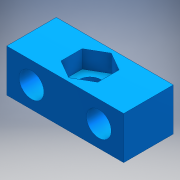
# Autodesk Inventor part: smallSprocketFixture
Saved by Autodesk Inventor 2016 (Build 200138000, 138)
## iProperties
Created: 2016-05-21
Part Number: smallSprocketFixture
Material: ABS Plastic
Document SubType Name: Modeling
Designer: Henrik Samuelsson
Density: 1.06 g/cm^3
Appearance: Smooth - White
Author: Henrik Samuelsson
Autodesk Inventor part; units mm, degrees
ref_plane "YZ Plane" through (0, 0, 0) normal (1, 0, 0) x (0, 1, 0)
ref_plane "XZ Plane" through (0, 0, 0) normal (0, 1, 0) x (-1, 0, 0)
ref_plane "XY Plane" through (0, 0, 0) normal (0, 0, 1) x (1, 0, 0)
sketch "Sketch1" plane through (0, 0, 0) normal (0, 1, 0) x (-1, 0, 0)
  line L0 (0, 0) -> (33, 0)
  line L1 (33, 0) -> (33, -12)
  line L2 (33, -12) -> (0, -12)
  line L3 (0, -12) -> (0, 0)
  circle A0 centre (26, -6) radius 3.5
  circle A1 centre (7, -6) radius 3.5
  dimension "d0" = 12
  dimension "d1" = 33
  dimension "d2" = 7
  dimension "d3" = 7
  dimension "d4" = 7
  dimension "d6" = 6
  dimension "d7" = 6
  dimension "d9" = 19
  constraints: 8 end point, 2 centre point, 2 parallel, 1 horizontal, 1 perpendicular
  measures "d0" distance of L1.end L0.end
  measures "d1" distance of L2.end L1.end
  measures "d2" diameter of A0
  measures "d3" diameter of A1
  measures "d4" distance from line of L1 A0.centre
  measures "d6" distance from line of L2 A1.centre
  measures "d7" distance from line of L2 A0.centre
  measures "d9" distance of A0.centre A1.centre
extrude "Extrusion1" add sketch "Sketch1" along normal mid plane 14
sketch "Sketch2" plane through (0, -7, -12) normal (0, 0, -1) x (-1, 0, 0)
  circle A0 centre (16.5, 7) radius 3.1
  line L0 (33, 14) -> (33, 0) projected
  line L1 (33, 0) -> (0, 0) projected
  point P0 (0, 7)
  dimension "d12" = 6.2
  dimension "d14" = 16.5
  dimension "d20" = 7
  constraints: 1 centre point
  measures "d12" diameter of A0
  measures "d14" distance from line of L0 A0.centre
  measures "d20" distance from line of L1 A0.centre
extrude "Extrusion2" cut sketch "Sketch2" against normal up to next
sketch "Sketch3" plane through (-33, -7, 0) normal (0, 0, 1) x (1, 0, 0)
  circle A0 centre (16.5, 7) radius 3.1 projected
  line L0 (16.5, 13.0044) -> (21.7, 10.0022)
  line L1 (21.7, 10.0022) -> (21.7, 3.9978)
  line L2 (21.7, 3.9978) -> (16.5, 0.9956)
  line L3 (16.5, 0.9956) -> (11.3, 3.9978)
  line L4 (11.3, 3.9978) -> (11.3, 10.0022)
  line L5 (11.3, 10.0022) -> (16.5, 13.0044)
  line L6 (0, 14) -> (33, 14) projected
  line L7 (0, 14) -> (0, 0) projected
  point P0 (33, 7)
  dimension "d17" = 5.2
  constraints: 12 end point, 1 coincident, 1 parallel, 12 other
  measures "d17" distance from line of L5 point (16.5, 7)
extrude "Extrusion3" cut sketch "Sketch3" against normal blind 5
body "Solid1"
